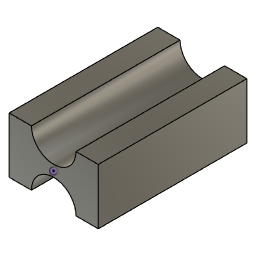
Tutorial Part 2 v2 (Autodesk Fusion 360 design; units mm, degrees)
Autodesk Fusion 360 part; units mm, degrees
sketch "Sketch1" plane through (0, 0, 0) normal (0, 0, 1) x (1, 0, 0)
sketch "Sketch2" plane through (0, 0, 0) normal (0, 1, 0) x (1, 0, 0)
  line L0 (24, -15) -> (-24, -15)
  line L1 (-24, -15) -> (-24, 15)
  line L2 (-24, 15) -> (24, 15)
  line L3 (24, 15) -> (24, -15)
  line L4 (24, -15) -> (-24, 15) construction
  line L5 (-24, -15) -> (24, 15) construction
  dimension "d3" = 48
  dimension "d4" = 30
  constraint horizontal L0
  constraint perpendicular L0 L1
  constraint parallel L0 L2
  constraint parallel L1 L3
  constraint coincident L4 origin
  constraint coincident L5 origin
  measures "d3" distance of L1.end L2.end
  measures "d4" distance of L0.start L2.end
extrude "Extrude1" add sketch "Sketch2" along normal blind 80
sketch "Sketch3" plane through (0, 0, 0) normal (0, -1, 0) x (1, 0, 0)
  line L0 (-24, -15) -> (24, -15)
  line L1 (24, -15) -> (24, 15)
  line L2 (24, 15) -> (-24, 15)
  line L3 (-24, 15) -> (-24, -15)
  arc A0 (-12, 15) -> (12, 15) centre (0, 15) ccw
  arc A1 (12, -15) -> (-12, -15) centre (0, -15) ccw
  line L4 (-12, -15) -> (12, -15)
  line L5 (12, 15) -> (-12, 15)
  dimension "d7" = 12
  dimension "d8" = 12
  constraint coincident L2 A0.start
  constraint midpoint L2 A0.centre
  constraint coincident L0 A1.end
  constraint midpoint L0 A1.centre
  constraint parallel L0 L4
  constraint parallel L2 L5
  measures "d7" radius of A0
  measures "d8" radius of A1
extrude "Extrude2" cut sketch "Sketch3" against normal blind 80 contours L0 A1 L4 | L2 A0 L5
